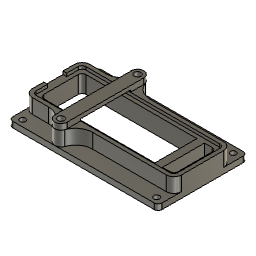
ESP-PROGHolder (Autodesk Fusion 360 design; units mm, degrees)
Autodesk Fusion 360 part; units mm, degrees
sketch "Sketch1" plane through (0, 0, 0) normal (0, 0, 1) x (1, 0, 0) in component "ESP-ProgHolder"
  line L0 (39, 15) -> (-39, 15)
  line L1 (-39, 15) -> (-39, -15)
  line L2 (-39, -15) -> (39, -15)
  line L3 (39, -15) -> (39, 15)
  line L4 (39, 15) -> (-39, -15) construction
  line L5 (-39, 15) -> (39, -15) construction
  dimension "d4" = 78
  dimension "d5" = 30
  constraint horizontal L0
  constraint perpendicular L0 L1
  constraint parallel L0 L2
  constraint parallel L1 L3
  constraint coincident L4 origin
  constraint coincident L5 origin
  measures "d4" distance of L1.end L2.end
  measures "d5" distance of L0.end L1.end
extrude "Extrude1" add sketch "Sketch1" along normal blind 6 makes body 1 in component "ESP-ProgHolder"
sketch "Sketch2" plane through (0, 0, 6) normal (0, 0, 1) x (-1, 0, 0) in component "ESP-ProgHolder"
  line L0 (-39, 15) -> (-39, -15)
  line L1 (-39, -15) -> (39, -15)
  line L2 (39, -15) -> (39, 15)
  line L3 (39, 15) -> (-39, 15)
  line L4 (35, 11) -> (-35, 11)
  line L5 (-35, 11) -> (-35, -11)
  line L6 (-35, -11) -> (35, -11)
  line L7 (35, -11) -> (35, 11)
extrude "Extrude2" cut sketch "Sketch2" against normal up to surface (6 mm away) contours L4 L5 L6 L7 bodies 1 in component "ESP-ProgHolder"
fillet "Fillet1" radius 2 4 edges at (-35, 11, 3) (35, -11, 3) (-35, -11, 3) (35, 11, 3) on bodies 1 in component "ESP-ProgHolder"
fillet "Fillet2" radius 4 4 edges at (-39, -15, 3) (-39, 15, 3) (39, -15, 3) (39, 15, 3) on bodies 1 in component "ESP-ProgHolder"
sketch "Sketch3" plane through (0, 0, 6) normal (0, 0, 1) x (-1, 0, 0) in component "ESP-ProgHolder"
  arc A0 (-39, -11) -> (-35, -15) centre (-35, -11) ccw
  line L0 (-35, -15) -> (35, -15)
  arc A1 (35, -15) -> (39, -11) centre (35, -11) ccw
  line L1 (39, -11) -> (39, 11)
  arc A2 (39, 11) -> (35, 15) centre (35, 11) ccw
  line L2 (35, 15) -> (-35, 15)
  arc A3 (-35, 15) -> (-39, 11) centre (-35, 11) ccw
  line L3 (-39, 11) -> (-39, -11)
  line L4 (33, -11) -> (-33, -11)
  arc A4 (-35, -9) -> (-33, -11) centre (-33, -9) ccw
  line L5 (-35, -9) -> (-35, 9)
  arc A5 (-33, 11) -> (-35, 9) centre (-33, 9) ccw
  line L6 (-33, 11) -> (33, 11)
  arc A6 (35, 9) -> (33, 11) centre (33, 9) ccw
  line L7 (35, 9) -> (35, -9)
  arc A7 (33, -11) -> (35, -9) centre (33, -9) ccw
  line L8 (-37, 11) -> (-37, -11)
  arc A8 (-37, -11) -> (-35, -13) centre (-35, -11) ccw
  line L9 (-35, -13) -> (35, -13)
  arc A9 (35, -13) -> (37, -11) centre (35, -11) ccw
  line L10 (37, -11) -> (37, 11)
  arc A10 (37, 11) -> (35, 13) centre (35, 11) ccw
  line L11 (35, 13) -> (-35, 13)
  arc A11 (-35, 13) -> (-37, 11) centre (-35, 11) ccw
  dimension "d17" = -2
extrude "Extrude3" add sketch "Sketch3" along normal blind 1.6 contours A0 L0 A1 L1 A2 L2 A3 L3 bodies 1 in component "ESP-ProgHolder"
sketch "Sketch4" plane through (-39, 0, 0) normal (-1, 0, 0) x (0, -1, 0) in component "ESP-ProgHolder"
  line L0 (-11, 7.6) -> (-11, 0)
  line L1 (-11, 0) -> (11, 0)
  line L2 (11, 0) -> (11, 7.6)
  line L3 (11, 7.6) -> (-11, 7.6)
  line L4 (-5, 7.6) -> (5, 7.6)
  line L5 (5, 7.6) -> (5, 6)
  line L6 (5, 6) -> (-5, 6)
  line L7 (-5, 6) -> (-5, 7.6)
  line L8 (-5, 7.6) -> (5, 6) construction
  line L9 (5, 7.6) -> (-5, 6) construction
  point P0 (0, 6.8)
  dimension "d20" = 10
  dimension "d21" = 1.6
  constraint horizontal L4
  constraint perpendicular L4 L5
  constraint parallel L4 L6
  constraint parallel L5 L7
  constraint coincident L8 P0
  constraint coincident L9 P0
  constraint collinear L3 L4
  measures "d20" distance of L5.end L6.end
  measures "d21" distance of L4.end L5.end
extrude "Extrude4" cut sketch "Sketch4" against normal up to surface (2 mm away) contours L3 L4 L5 L6 L7 bodies 1 in component "ESP-ProgHolder"
sketch "Sketch7" plane through (0, 11, 0) normal (0, -1, 0) x (1, 0, 0) in component "ESP-ProgHolder"
  line L0 (33, 0) -> (33, 6)
  line L1 (33, 6) -> (-33, 6)
  line L2 (-33, 6) -> (-33, 0)
  line L3 (-33, 0) -> (33, 0)
  line L4 (25, 6) -> (29, 6)
  line L5 (29, 6) -> (29, 0)
  line L6 (29, 0) -> (25, 0)
  line L7 (25, 0) -> (25, 6)
  line L8 (35, 7.6) -> (35, 0)
  dimension "d24" = 4
  dimension "d25" = 6
  dimension "d26" = 6
  constraint horizontal L4
  constraint vertical L5
  constraint horizontal L6
  constraint vertical L7
  constraint coincident L1 L4.start
  measures "d24" distance of L4.start L4.end
  measures "d25" distance of L4.start L6.end
  measures "d26" distance of L4.end L8
extrude "Extrude5" add sketch "Sketch7" along normal up to surface (22 mm away) contours L1 L3 L4 L5 L6 L7 bodies 1 in component "ESP-ProgHolder"
sketch "Sketch14" plane through (0, 0, 7.6) normal (0, 0, 1) x (-1, 0, 0) in component "ESP-ProgHolder"
  line L0 (37, 5) -> (39, 5)
  line L1 (39, 5) -> (39, 11)
  arc A0 (39, 11) -> (35, 15) centre (35, 11) ccw
  line L2 (35, 15) -> (-35, 15)
  arc A1 (-35, 15) -> (-39, 11) centre (-35, 11) ccw
  line L3 (-39, 11) -> (-39, -11)
  arc A2 (-39, -11) -> (-35, -15) centre (-35, -11) ccw
  line L4 (-35, -15) -> (35, -15)
  arc A3 (35, -15) -> (39, -11) centre (35, -11) ccw
  line L5 (39, -11) -> (39, -5)
  line L6 (39, -5) -> (37, -5)
  line L7 (37, -5) -> (37, -11)
  arc A4 (35, -13) -> (37, -11) centre (35, -11) ccw
  line L8 (35, -13) -> (-35, -13)
  arc A5 (-37, -11) -> (-35, -13) centre (-35, -11) ccw
  line L9 (-37, -11) -> (-37, 11)
  arc A6 (-35, 13) -> (-37, 11) centre (-35, 11) ccw
  line L10 (-35, 13) -> (35, 13)
  arc A7 (37, 11) -> (35, 13) centre (35, 11) ccw
  line L11 (37, 11) -> (37, 5)
  line L12 (15, -20) -> (15, 20) construction
  circle A8 centre (15, -20) radius 3.25
  circle A9 centre (15, -20) radius 1.75
  circle A10 centre (15, 20) radius 3.25
  circle A11 centre (15, 20) radius 1.75
  line L13 (-43, 0) -> (50, 0) construction
  line L14 (18.25, -20) -> (18.25, -15)
  line L15 (11.75, -20) -> (11.75, -15)
  line L16 (11.75, 20) -> (11.75, 15)
  line L17 (18.25, 20) -> (18.25, 15)
  dimension "d104" = 22
  dimension "d105" = 6.5
  dimension "d106" = 3.5
  dimension "d107" = 6.5
  dimension "d108" = 3.5
  dimension "d216" = 20
  dimension "d217" = 20
  constraint concentric A8 A9
  constraint concentric A10 A11
  constraint coincident L12 A8.centre
  constraint coincident L12 A10.centre
  constraint horizontal L13
  constraint coincident A8 L14.start
  constraint coincident L4 L14.end
  constraint tangent A8 L14
  constraint coincident A8 L15.start
  constraint coincident L4 L15.end
  constraint tangent A8 L15
  constraint perpendicular L4 L15
  constraint perpendicular L4 L14
  constraint coincident A10 L16.start
  constraint coincident L2 L16.end
  constraint tangent A10 L16
  constraint coincident A10 L17.start
  constraint coincident L2 L17.end
  constraint tangent A10 L17
  constraint perpendicular L2 L16
  constraint perpendicular L2 L17
  measures "d104" distance of L7 L12
  measures "d105" diameter of A8
  measures "d106" diameter of A9
  measures "d107" diameter of A10
  measures "d108" diameter of A11
  measures "d216" distance of L12.start L13
  measures "d217" distance of L12.end L13
extrude "Extrude11" add sketch "Sketch14" against normal up to surface (7.6 mm away) contours L4 A8 L14 L15 bodies 1 in component "ESP-ProgHolder"
extrude "Extrude12" add sketch "Sketch14" against normal up to surface (7.6 mm away) contours L2 A10 L16 L17 bodies 1 in component "ESP-ProgHolder"
extrude "Extrude13" cut sketch "Sketch14" against normal up to surface (7.6 mm away) contours A9 | A11 bodies 1 in component "ESP-ProgHolder"
extrude "Extrude14" add sketch "Sketch14" against normal up to surface (7.6 mm away) contours A10 bodies 1 in component "ESP-ProgHolder"
extrude "Extrude15" add sketch "Sketch14" against normal up to surface (7.6 mm away) contours A8 bodies 1 in component "ESP-ProgHolder"
fillet "Fillet4" radius 9 4 edges at (-18.25, -15, 3.8) (-11.75, -15, 3.8) (-11.75, 15, 3.8) (-18.25, 15, 3.8) on bodies 1 in component "ESP-ProgHolder"
sketch "Sketch1 (2)" plane through (0, 0, 7.6) normal (0, 0, 1) x (-1, 0, 0) in component "ESP-Clamp"
  circle A0 centre (15, -20) radius 1.75
  circle A1 centre (15, 20) radius 1.75
  line L0 (37, 5) -> (39, 5)
  line L1 (39, 5) -> (39, 11)
  arc A2 (39, 11) -> (35, 15) centre (35, 11) ccw
  line L2 (35, 15) -> (26.5785, 15)
  arc A3 (18.0719, 21.0612) -> (26.5785, 15) centre (26.5785, 24) ccw
  arc A4 (18.0719, 21.0612) -> (11.9281, 21.0612) centre (15, 20) ccw
  arc A5 (3.4215, 15) -> (11.9281, 21.0612) centre (3.4215, 24) ccw
  line L3 (3.4215, 15) -> (-35, 15)
  arc A6 (-35, 15) -> (-39, 11) centre (-35, 11) ccw
  line L4 (-39, 11) -> (-39, -11)
  arc A7 (-39, -11) -> (-35, -15) centre (-35, -11) ccw
  line L5 (-35, -15) -> (3.4215, -15)
  arc A8 (11.9281, -21.0612) -> (3.4215, -15) centre (3.4215, -24) ccw
  arc A9 (11.9281, -21.0612) -> (18.0719, -21.0612) centre (15, -20) ccw
  arc A10 (26.5785, -15) -> (18.0719, -21.0612) centre (26.5785, -24) ccw
  line L6 (26.5785, -15) -> (35, -15)
  arc A11 (35, -15) -> (39, -11) centre (35, -11) ccw
  line L7 (39, -11) -> (39, -5)
  line L8 (39, -5) -> (37, -5)
  line L9 (37, -5) -> (37, -11)
  arc A12 (35, -13) -> (37, -11) centre (35, -11) ccw
  line L10 (35, -13) -> (-35, -13)
  arc A13 (-37, -11) -> (-35, -13) centre (-35, -11) ccw
  line L11 (-37, -11) -> (-37, 11)
  arc A14 (-35, 13) -> (-37, 11) centre (-35, 11) ccw
  line L12 (-35, 13) -> (35, 13)
  arc A15 (37, 11) -> (35, 13) centre (35, 11) ccw
  line L13 (37, 11) -> (37, 5)
  arc A16 (11.9281, -21.0612) -> (18.0719, -21.0612) centre (15, -20) ccw
  arc A17 (18.0719, 21.0612) -> (11.9281, 21.0612) centre (15, 20) ccw
  circle A18 centre (15, -20) radius 1.75
  circle A19 centre (15, -20) radius 3.25
  circle A20 centre (15, 20) radius 1.75
  circle A21 centre (15, 20) radius 3.25
  line L14 (11.75, -20) -> (11.75, 20)
  line L15 (18.25, -20) -> (18.25, 20)
  constraint concentric A16 A18
  constraint concentric A16 A19
  constraint coincident A8.start A19
  constraint concentric A17 A20
  constraint concentric A17 A21
  constraint coincident A4.end A21
  constraint coincident A19 L14.start
  constraint coincident A21 L14.end
  constraint tangent A21 L14
  constraint coincident A19 L15.start
  constraint coincident A21 L15.end
  constraint tangent A21 L15
  constraint tangent A19 L15
  constraint tangent A19 L14
extrude "Extrude1'" add sketch "Sketch1 (2)" along normal blind 3 separate body contours L10 L12 L14 L15 | L12 A21 L14 L15 | L10 A19 L14 L15 | A4 A17 A21 | A9 A16 A19 makes body 2 in component "ESP-Clamp"
sketch "Sketch2 (2)" plane through (0, 0, 7.6) normal (0, 0, -1) x (1, 0, 0) in component "ESP-Clamp"
  circle A0 centre (-15, -20) radius 1.75
  circle A1 centre (-15, 20) radius 1.75
  arc A2 (-18.25, -20) -> (-11.75, -20) centre (-15, -20) ccw
  line L0 (-11.75, -20) -> (-11.75, 20)
  arc A3 (-11.75, 20) -> (-18.25, 20) centre (-15, 20) ccw
  line L1 (-18.25, 20) -> (-18.25, -20)
  line L2 (-18.25, 13) -> (-11.75, 13)
  line L3 (-11.75, 13) -> (-11.75, -13)
  line L4 (-11.75, -13) -> (-18.25, -13)
  line L5 (-18.25, -13) -> (-18.25, 13)
  line L6 (-35, 13) -> (35, 13)
  line L7 (35, -13) -> (-35, -13)
  constraint horizontal L2
  constraint vertical L3
  constraint horizontal L4
  constraint vertical L5
  constraint coincident L0 L3.end
  constraint coincident L1 L2.start
  constraint coincident L2.start L6
  constraint coincident L4.end L7
extrude "Extrude2'" cut sketch "Sketch2 (2)" against normal blind 1 contours L0 L1 L2 L3 L4 L5 L6 L7 bodies 2 in component "ESP-Clamp"
sketch "Sketch7 (2)" plane through (0, 0, 0) normal (0, 0, -1) x (1, 0, 0)
  circle A0 centre (-15, -20) radius 1.75
  circle A1 centre (-15, 20) radius 1.75
  line L0 (25, -11) -> (-33, -11)
  arc A2 (-35, -9) -> (-33, -11) centre (-33, -9) ccw
  line L1 (-35, -9) -> (-35, 9)
  arc A3 (-33, 11) -> (-35, 9) centre (-33, 9) ccw
  line L2 (-33, 11) -> (25, 11)
  line L3 (25, 11) -> (25, -11)
  line L4 (29, -11) -> (29, 11)
  line L5 (29, 11) -> (33, 11)
  arc A4 (35, 9) -> (33, 11) centre (33, 9) ccw
  line L6 (35, 9) -> (35, -9)
  arc A5 (33, -11) -> (35, -9) centre (33, -9) ccw
  line L7 (33, -11) -> (29, -11)
  arc A6 (35, -15) -> (39, -11) centre (35, -11) ccw
  line L8 (39, -11) -> (39, 11)
  arc A7 (39, 11) -> (35, 15) centre (35, 11) ccw
  line L9 (35, 15) -> (-3.4215, 15)
  arc A8 (-11.9281, 21.0612) -> (-3.4215, 15) centre (-3.4215, 24) ccw
  arc A9 (-11.9281, 21.0612) -> (-18.0719, 21.0612) centre (-15, 20) ccw
  arc A10 (-26.5785, 15) -> (-18.0719, 21.0612) centre (-26.5785, 24) ccw
  line L10 (-26.5785, 15) -> (-35, 15)
  arc A11 (-35, 15) -> (-39, 11) centre (-35, 11) ccw
  line L11 (-39, 11) -> (-39, -11)
  arc A12 (-39, -11) -> (-35, -15) centre (-35, -11) ccw
  line L12 (-35, -15) -> (-26.5785, -15)
  arc A13 (-18.0719, -21.0612) -> (-26.5785, -15) centre (-26.5785, -24) ccw
  arc A14 (-18.0719, -21.0612) -> (-11.9281, -21.0612) centre (-15, -20) ccw
  arc A15 (-3.4215, -15) -> (-11.9281, -21.0612) centre (-3.4215, -24) ccw
  line L13 (-3.4215, -15) -> (35, -15)
  line L14 (-39, 23.25) -> (39, 23.25)
  line L15 (39, 23.25) -> (39, -23.25)
  line L16 (39, -23.25) -> (-39, -23.25)
  line L17 (-39, -23.25) -> (-39, 23.25)
  line L18 (-39, 23.25) -> (39, -23.25) construction
  line L19 (39, 23.25) -> (-39, -23.25) construction
  constraint horizontal L14
  constraint perpendicular L14 L15
  constraint parallel L14 L16
  constraint parallel L15 L17
  constraint coincident L18 origin
  constraint coincident L19 origin
  constraint tangent A9 L14
  constraint collinear L11 L17
extrude "Extrude16" add sketch "Sketch7 (2)" along normal blind 3 bodies 1 in component "ESP-ProgHolder"
fillet "Fillet5" radius 2 4 edges at (-39, -23.25, -1.5) (39, -23.25, -1.5) (39, 23.25, -1.5) (-39, 23.25, -1.5) on bodies 1 in component "ESP-ProgHolder"
sketch "Sketch8" plane through (0, 0, 0) normal (0, 0, 1) x (-1, 0, 0)
  arc A0 (37, -23.25) -> (39, -21.25) centre (37, -21.25) ccw
  line L0 (39, -21.25) -> (39, -11)
  arc A1 (35, -15) -> (39, -11) centre (35, -11) ccw
  line L1 (35, -15) -> (26.5785, -15)
  arc A2 (26.5785, -15) -> (18.0719, -21.0612) centre (26.5785, -24) ccw
  arc A3 (15, -23.25) -> (18.0719, -21.0612) centre (15, -20) ccw
  line L2 (15, -23.25) -> (37, -23.25)
  circle A4 centre (35, -20) radius 1.5
  circle A5 centre (-35, -20) radius 1.5
  circle A6 centre (35, 20) radius 1.5
  circle A7 centre (-35, 20) radius 1.5
  dimension "d232" = 3
  dimension "d233" = 3.25
  dimension "d234" = 4
  dimension "d237" = -70
  dimension "d238" = 40
  measures "d232" diameter of A4
  measures "d233" distance of L2 A4.centre
  measures "d234" distance of L0 A4.centre
extrude "Extrude17" cut sketch "Sketch8" against normal up to surface (3 mm away) contours A4 | A5 | A6 | A7 bodies 1 in component "ESP-ProgHolder"
component "ESP-ProgHolder" placed x (1, 0, 0) y (0, 1, 0) z (0, 0, 1) at (0, 0, 0)
component "ESP-Clamp" placed x (1, 0, 0) y (0, 1, 0) z (0, 0, 1) at (0, 0, 0)
equation "ESPProgLength = 73.5 mm"
equation "ESPProgWidth = 27 mm"
equation "ESPProgPCBHeight = 1.6 mm"
equation "d4 = ESPProgLength + 4.5 mm"
equation "d5 = ESPProgWidth + SupportWidth - 1 mm"
equation "d6 = SupportHeight"
equation "d8 = -SupportWidth"
equation "SupportHeight = 6 mm"
equation "SupportWidth = 4 mm"
equation "d17 = -( SupportWidth / 2 )"
equation "d18 = ESPProgPCBHeight"
equation "d21 = ESPProgPCBHeight"
equation "d25 = SupportHeight"
equation "STLinkWidth = 15.5 mm"
equation "STLinkLength = 29 mm"
equation "STLinkHeight = 1.75 mm"
equation "STLinkPlugWidth = 4 mm"
equation "STLinkPlugHeight = 8 mm"
equation "STLinkPlugLength = 13.5 mm"
equation "STLinkPlugCableWidth = 10 mm"
equation "STLinkBaseHeight = 0 mm"
equation "STLinkSupportHeight = STLinkPlugHeight + 1 mm"
equation "d105 = d106 + 3 mm"
equation "d106 = ScrewDiameter"
equation "d107 = d108 + 3 mm"
equation "d108 = ScrewDiameter"
equation "ScrewDiameter = 3.5 mm"
equation "PogoboardScrewDiameter = 3 mm"
equation "PogoboardSupportHeight = 10 mm"
equation "EmbeddedBreakoutSupportHeight = 6 mm"
